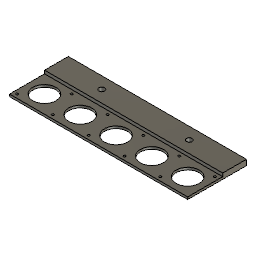
Pumpenhalterung (Autodesk Fusion 360 design; units mm, degrees)
part number: 2025-11-29-22-39-40-542
Autodesk Fusion 360 part; units mm, degrees
note: some values were not read from the file. Chosen so that the rebuilt part matches the saved one: which bodies a step acts on; which face or edge a step refers to. Set by a fixed rule: which sketch regions a step uses.
sketch "Skizze1" plane through (0, 0, 0) normal (0, 0, 1) x (1, 0, 0)
  line L0 (0, 0) -> (200, 0)
  line L1 (200, 0) -> (200, 70)
  line L2 (200, 70) -> (0, 70)
  line L3 (0, 70) -> (0, 0)
  dimension "d1" = 200
  dimension "d2" = 70
  constraint horizontal L0
  constraint vertical L1
  constraint horizontal L2
  constraint vertical L3
  constraint coincident L0.start L3.end
  measures "d1" distance of L0.start L0.end
  measures "d2" distance of L0.start L2.end
extrude "Extrusion1" add sketch "Skizze1" along normal blind 3 makes body 1
sketch "Skizze2" plane through (0, 0, 3) normal (0, 0, 1) x (-1, 0, 0)
  line L0 (0, -70) -> (0, 0)
  line L1 (0, 0) -> (-200, 0)
  line L2 (-200, 0) -> (-200, -70)
  line L3 (-200, -70) -> (0, -70)
  line L4 (0, -70) -> (-200, -70)
  line L5 (-200, -70) -> (-200, -40)
  line L6 (-200, -40) -> (0, -40)
  line L7 (0, -40) -> (0, -70)
  dimension "d5" = 30
  constraint horizontal L4
  constraint vertical L5
  constraint horizontal L6
  constraint vertical L7
  constraint coincident L0.start L3.end
  measures "d5" distance of L0.start L6.end
extrude "Extrusion2" add sketch "Skizze2" along normal blind 4 contours L0 L2 L3 L4 L5 L6 L7 bodies 1
sketch "Skizze3" plane through (0, 0, 7) normal (0, 0, 1) x (-1, 0, 0)
  line L0 (0, -40) -> (-200, -40)
  line L1 (-200, -40) -> (-200, -70)
  line L2 (-200, -70) -> (0, -70)
  line L3 (0, -70) -> (0, -40)
  line L4 (0, -55) -> (-200, -55)
  line L5 (-100, -55) -> (-100, -70)
  circle A0 centre (-50, -55) radius 3.5
  circle A1 centre (-150, -55) radius 3.5
  dimension "d8" = 7
  dimension "d9" = 7
  constraint midpoint L3 L4.start
  constraint midpoint L1 L4.end
  constraint midpoint L4 L5.start
  constraint midpoint L2 L5.end
  constraint coincident L4 A0.centre
  constraint coincident L4 A1.centre
  measures "d8" diameter of A0
  measures "d9" diameter of A1
extrude "Extrusion3" cut sketch "Skizze3" against normal blind 15 contours L4 A0 | L4 A0 | L4 A1 | L4 A1 bodies 1
sketch "Skizze4" plane through (0, 0, 3) normal (0, 0, 1) x (-1, 0, 0)
  line L0 (-200, -40) -> (0, -40)
  line L1 (0, -40) -> (0, 0)
  line L2 (0, 0) -> (-200, 0)
  line L3 (-200, 0) -> (-200, -40)
  circle A0 centre (-20, -20) radius 14.5
  circle A1 centre (-60, -20) radius 14.5
  circle A2 centre (-100, -20) radius 14.5
  circle A3 centre (-140, -20) radius 14.5
  circle A4 centre (-180, -20) radius 14.5
  dimension "d12" = 29
  dimension "d13" = 29
  dimension "d14" = 29
  dimension "d15" = 29
  dimension "d16" = 29
  measures "d12" diameter of A0
  measures "d13" diameter of A1
  measures "d14" diameter of A2
  measures "d15" diameter of A3
  measures "d16" diameter of A4
extrude "Extrusion4" cut sketch "Skizze4" against normal blind 10 contours A0 | A1 | A2 | A3 | A4 bodies 1
sketch "Skizze5" plane through (0, 0, 3) normal (0, 0, 1) x (-1, 0, 0)
  circle A0 centre (-100, -20) radius 14.5
  circle A1 centre (-60, -20) radius 14.5
  circle A2 centre (-140, -20) radius 14.5
  circle A3 centre (-20, -20) radius 14.5
  circle A4 centre (-180, -20) radius 14.5
  line L0 (-200, -40) -> (0, -40)
  line L1 (0, -40) -> (0, 0)
  line L2 (0, 0) -> (-200, 0)
  line L3 (-200, 0) -> (-200, -40)
  line L4 (-20, -20) -> (-37.1827, -37.1827)
  line L5 (-20, -20) -> (4.3, -20) construction
  line L6 (-20, -20) -> (-2.8173, -2.8173)
  line L7 (-60, -20) -> (-77.1827, -37.1827)
  line L8 (-60, -20) -> (-35.7, -20) construction
  line L9 (-42.8173, -2.8173) -> (-60, -20)
  line L10 (-100, -20) -> (-117.1827, -37.1827)
  line L11 (-100, -20) -> (-75.7, -20) construction
  line L12 (-100, -20) -> (-82.8173, -2.8173)
  line L13 (-140, -20) -> (-157.1827, -37.1827)
  line L14 (-140, -20) -> (-115.7, -20) construction
  line L15 (-140, -20) -> (-122.8173, -2.8173)
  line L16 (-180, -20) -> (-197.1827, -37.1827)
  line L17 (-180, -20) -> (-162.8173, -2.8173)
  circle A5 centre (-2.8173, -2.8173) radius 1.4
  circle A6 centre (-37.1827, -37.1827) radius 1.4
  circle A7 centre (-42.8173, -2.8173) radius 1.4
  circle A8 centre (-77.1827, -37.1827) radius 1.4
  circle A9 centre (-82.8173, -2.8173) radius 1.4
  circle A10 centre (-117.1827, -37.1827) radius 1.4
  circle A11 centre (-122.8173, -2.8173) radius 1.4
  circle A12 centre (-157.1827, -37.1827) radius 1.4
  circle A13 centre (-162.8173, -2.8173) radius 1.4
  circle A14 centre (-197.1827, -37.1827) radius 1.4
  dimension "d19" = 135
  dimension "d20" = 24.3
  dimension "d21" = 24.3
  dimension "d22" = 135
  dimension "d23" = 24.3
  dimension "d24" = 135
  dimension "d25" = 24.3
  dimension "d26" = 24.3
  dimension "d27" = 135
  dimension "d28" = 24.3
  dimension "d29" = 24.3
  dimension "d30" = 24.3
  dimension "d31" = 24.3
  dimension "d32" = 2.8
  dimension "d33" = 2.8
  dimension "d34" = 2.8
  dimension "d35" = 2.8
  dimension "d36" = 2.8
  dimension "d37" = 2.8
  dimension "d38" = 2.8
  dimension "d39" = 2.8
  dimension "d40" = 2.8
  dimension "d41" = 2.8
  constraint horizontal L5
  constraint coincident A3.centre L4.start
  constraint parallel L4 L6
  constraint horizontal L8
  constraint coincident A1.centre L7.start
  constraint parallel L7 L9
  constraint horizontal L11
  constraint coincident A0.centre L10.start
  constraint parallel L10 L12
  constraint horizontal L14
  constraint coincident A2.centre L13.start
  constraint parallel L13 L15
  constraint coincident A4.centre L16.start
  constraint parallel L16 L17
  constraint coincident L6.end A5.centre
  constraint coincident L4.end A6.centre
  constraint coincident L9.start A7.centre
  constraint coincident L7.end A8.centre
  constraint coincident L12.end A9.centre
  constraint coincident L10.end A10.centre
  constraint coincident L15.end A11.centre
  constraint coincident L13.end A12.centre
  constraint coincident L17.end A13.centre
  constraint coincident L16.end A14.centre
  measures "d19" angle of L4 L5
  measures "d20" distance of A3.centre L4.end
  measures "d21" distance of A3.centre L6.end
  measures "d22" angle of L7 L8
  measures "d23" distance of A1.centre L7.end
  measures "d24" angle of L10 L11
  measures "d25" distance of A0.centre L10.end
  measures "d26" distance of A0.centre L12.end
  measures "d27" angle of L13 L14
  measures "d28" distance of A2.centre L13.end
  measures "d29" distance of A2.centre L15.end
  measures "d30" distance of A4.centre L16.end
  measures "d31" distance of A4.centre L17.end
  measures "d32" diameter of A5
  measures "d33" diameter of A6
  measures "d34" diameter of A7
  measures "d35" diameter of A8
  measures "d36" diameter of A9
  measures "d37" diameter of A10
  measures "d38" diameter of A11
  measures "d39" diameter of A12
  measures "d40" diameter of A13
  measures "d41" diameter of A14
extrude "Extrusion5" cut sketch "Skizze5" against normal blind 7 contours A5 | A6 | A7 | A8 | A9 | A10 | A11 | A12 | A13 | A14 bodies 1
split "Teilen1" by plane through (200, 40, 3) normal (0, -1, 0) bodies 1 makes body 2 at (40.7452, 10.5027, 0)
move_body "Verschieben1" bodies 2 to x (1, 0, 0) y (0, 1, 0) z (0, 0, 1) at (0, -2, 0)
sketch "Skizze6" plane through (0, 0, 3) normal (0, 0, 1) x (-1, 0, 0)
  circle A0 centre (-157.1827, -35.1827) radius 1.4
  circle A1 centre (-77.1827, -35.1827) radius 1.4
  circle A2 centre (-37.1827, -35.1827) radius 1.4
  circle A3 centre (-82.8173, -0.8173) radius 1.4
  circle A4 centre (-197.1827, -35.1827) radius 1.4
  circle A5 centre (-122.8173, -0.8173) radius 1.4
  circle A6 centre (-42.8173, -0.8173) radius 1.4
  circle A7 centre (-2.8173, -0.8173) radius 1.4
  circle A8 centre (-117.1827, -35.1827) radius 1.4
  circle A9 centre (-162.8173, -0.8173) radius 1.4
  circle A10 centre (-100, -18) radius 14.5
  circle A11 centre (-60, -18) radius 14.5
  circle A12 centre (-140, -18) radius 14.5
  circle A13 centre (-20, -18) radius 14.5
  circle A14 centre (-180, -18) radius 14.5
  line L0 (-200, -38) -> (0, -38)
  line L1 (0, -38) -> (0, 2)
  line L2 (0, 2) -> (-200, 2)
  line L3 (-200, 2) -> (-200, -38)
  line L4 (0, -38) -> (-200, -38)
  line L5 (-200, -38) -> (-200, -40)
  line L6 (-200, -40) -> (0, -40)
  line L7 (0, -40) -> (0, -38)
  constraint horizontal L4
  constraint vertical L5
  constraint horizontal L6
  constraint vertical L7
  constraint coincident L0.end L1.start
extrude "Extrusion6" add sketch "Skizze6" against normal blind 3 contours L0 L4 L5 L6 L7 bodies 1 2
extrude "Extrusion7" add 1 faces at (66.6667, -2, 1) along direction (0, -1, 0) blind 2 on bodies 1 bodies 1
extrude "Extrusion8" add 1 faces at (0, 60, 3.3333) along direction (-1, 0, 0) blind 2 on bodies 1 bodies 1
extrude "Extrusion9" add 3 faces at (200, 10, 2) (200, 38.6667, 2) (200, 60, 3.3333) along direction (1, 0, 0) blind 2 on bodies 1 bodies 1
sketch "Skizze7" plane through (0, 0, 3) normal (0, 0, 1) x (-1, 0, 0)
  circle A0 centre (-157.1827, -35.1827) radius 1.4
  circle A1 centre (-77.1827, -35.1827) radius 1.4
  circle A2 centre (-37.1827, -35.1827) radius 1.4
  circle A3 centre (-82.8173, -0.8173) radius 1.4
  circle A4 centre (-197.1827, -35.1827) radius 1.4
  circle A5 centre (-122.8173, -0.8173) radius 1.4
  circle A6 centre (-42.8173, -0.8173) radius 1.4
  circle A7 centre (-2.8173, -0.8173) radius 1.4
  circle A8 centre (-117.1827, -35.1827) radius 1.4
  circle A9 centre (-162.8173, -0.8173) radius 1.4
  circle A10 centre (-100, -18) radius 14.5
  circle A11 centre (-60, -18) radius 14.5
  circle A12 centre (-140, -18) radius 14.5
  circle A13 centre (-20, -18) radius 14.5
  circle A14 centre (-180, -18) radius 14.5
  line L0 (2, 4) -> (-202, 4)
  line L1 (-202, 4) -> (-202, -38)
  line L2 (-202, -38) -> (-202, -40)
  line L3 (-202, -40) -> (-200, -40)
  line L4 (-200, -40) -> (2, -40)
  line L5 (2, -40) -> (2, 4)
  line L6 (0, 4) -> (-40, 4)
  line L7 (-40, 4) -> (-40, -40)
  line L8 (-40, 4) -> (-80, 4)
  line L9 (-80, 4) -> (-80, -40)
  line L10 (-80, 4) -> (-120, 4)
  line L11 (-120, -40) -> (-120, 4)
  line L12 (-120, 4) -> (-160, 4)
  line L13 (-160, 4) -> (-160, -40)
  constraint coincident L0 L6.start
  constraint coincident L0 L6.end
  constraint coincident L4 L7.end
  constraint perpendicular L4 L7
  constraint coincident L0 L8.end
  constraint coincident L4 L9.end
  constraint perpendicular L4 L9
  constraint coincident L0 L10.end
  constraint coincident L4 L11.start
  constraint perpendicular L0 L11
  constraint coincident L0 L12.end
  constraint coincident L4 L13.end
  constraint perpendicular L4 L13
split "Teilen2" by curves path "Skizze7" along L7 L9 L11 bodies 1 makes body 3 at (18.9721, 57.4865, 0) makes body 4 at (71.1667, 55, 0) makes body 5 at (100.3612, 57.4865, 0)
sketch "Skizze8" plane through (0, 0, 3) normal (0, 0, 1) x (-1, 0, 0)
  line L0 (-120, -40) -> (-120, 4)
  line L1 (-120, 4) -> (-202, 4)
  line L2 (-202, 4) -> (-202, -38)
  line L3 (-202, -38) -> (-202, -40)
  line L4 (-202, -40) -> (-200, -40)
  line L5 (-200, -40) -> (-120, -40)
  circle A0 centre (-157.1827, -35.1827) radius 1.4
  circle A1 centre (-197.1827, -35.1827) radius 1.4
  circle A2 centre (-122.8173, -0.8173) radius 1.4
  circle A3 centre (-162.8173, -0.8173) radius 1.4
  circle A4 centre (-140, -18) radius 14.5
  circle A5 centre (-180, -18) radius 14.5
  line L6 (-160, 4) -> (-160, -40)
  constraint coincident L1 L6.start
  constraint midpoint L5 L6.end
  constraint vertical L6
split "Teilen3" by curves path "Skizze8" along L6 bodies 1 makes body 6 at (181.0279, 57.4865, 0)
move_body "Verschieben2" bodies 6 to x (1, 0, 0) y (0, 1, 0) z (0, 0, 1) at (10, 0, 0)
move_body "Verschieben3" bodies 1 to x (1, 0, 0) y (0, 1, 0) z (0, 0, 1) at (5, 0, 0)
move_body "Verschieben4" bodies 3 to x (1, 0, 0) y (0, 1, 0) z (0, 0, 1) at (-10, 0, 0)
move_body "Verschieben5" bodies 4 to x (1, 0, 0) y (0, 1, 0) z (0, 0, 1) at (-5, 0, 0)
extrude "Extrusion10" add 2 faces at (30, 10.6667, 1) (30, 60, 3.3333) along direction (1, 0, 0) blind 5 on bodies 3 bodies 3 4
extrude "Extrusion11" add 1 faces at (75, 60, 3.3333) along direction (1, 0, 0) blind 5 on bodies 3 bodies 3 5
extrude "Extrusion12" add 1 faces at (120, 60, 3.3333) along direction (1, 0, 0) blind 5 on bodies 3 bodies 1 3
extrude "Extrusion13" add 1 faces at (165, 60, 3.3333) along direction (1, 0, 0) blind 5 on bodies 1 bodies 1 6
